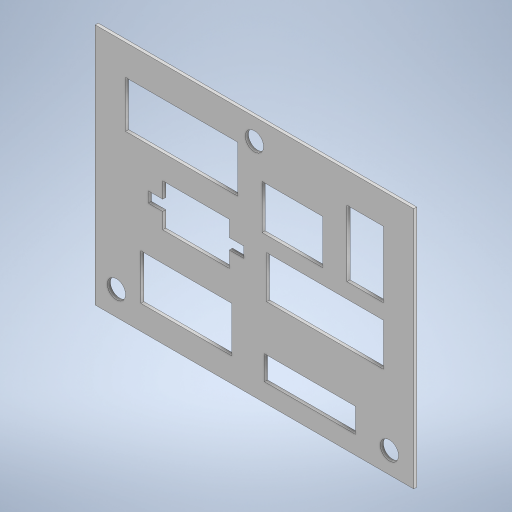
# Autodesk Inventor part: cap
Saved by Autodesk Inventor 2023 (Build 270158000, 158)
## iProperties
Created: 2023-04-07
Part Number: cap
Material: Generic
Document SubType Name: Sheet Metal
Designer: 310611102
Density: 1 g/cm^3
Sheet Metal Rule: Default_mm
Appearance: Default
Author: 310611102
Autodesk Inventor part; units mm, degrees
ref_plane "YZ Plane" through (0, 0, 0) normal (1, 0, 0) x (0, 1, 0)
ref_plane "XZ Plane" through (0, 0, 0) normal (0, 1, 0) x (-1, 0, 0)
ref_plane "XY Plane" through (0, 0, 0) normal (0, 0, 1) x (1, 0, 0)
sketch "Sketch1" plane through (0, 0, 0) normal (0, 0, 1) x (1, 0, 0)
  line L0 (-52.5, 40) -> (52.5, 40)
  line L1 (52.5, 40) -> (52.5, -40)
  line L2 (52.5, -40) -> (-52.5, -40)
  line L3 (-52.5, -40) -> (-52.5, 40)
  line L4 (-52.5, 40) -> (52.5, -40) construction
  line L5 (52.5, 40) -> (-52.5, -40) construction
  point P0 (0, 0)
  dimension "d0" = 80
  dimension "d1" = 105
  measures "d0" distance of L0.end L1.end
  measures "d1" distance of L0.start L0.end
extrude "Plate1" add sketch "Sketch1" along normal blind 1
sketch "Sketch3" plane through (0, 0, 0) normal (0, 0, -1) x (-1, 0, 0)
  line L0 (-42.5, 3.2) -> (-4, 3.2)
  line L1 (-4, 3.2) -> (-4, -10.8)
  line L2 (-4, -10.8) -> (-42.5, -10.8)
  line L3 (-42.5, -10.8) -> (-42.5, 3.2)
  line L4 (-42.5, 3.2) -> (-4, -10.8) construction
  line L5 (-4, 3.2) -> (-42.5, -10.8) construction
  line L6 (8.25, 6.6) -> (30.25, 6.6)
  line L7 (35, 1.35) -> (35, -2.15)
  line L8 (30.25, -7.4) -> (8.25, -7.4)
  line L9 (3.5, -2.15) -> (3.5, 1.35)
  line L10 (0.2073, 10) -> (38.2927, -10.8) construction
  line L11 (35, 6.6) -> (3.5, -7.4) construction
  line L12 (-2.5, 8.2) -> (-22.5, 8.2)
  line L13 (-22.5, 8.2) -> (-22.5, 22.8)
  line L14 (-22.5, 22.8) -> (-2.5, 22.8)
  line L15 (-2.5, 22.8) -> (-2.5, 8.2)
  line L16 (-2.5, 8.2) -> (-22.5, 22.8) construction
  line L17 (-22.5, 8.2) -> (-2.5, 22.8) construction
  line L18 (-3.29, -34) -> (-33.29, -34)
  line L19 (-33.29, -34) -> (-33.29, -26)
  line L20 (-33.29, -26) -> (-3.29, -26)
  line L21 (-3.29, -26) -> (-3.29, -34)
  line L22 (-3.29, -34) -> (-33.29, -26) construction
  line L23 (-33.29, -34) -> (-3.29, -26) construction
  line L24 (52.5, 40) -> (-52.5, 40) projected
  line L25 (52.5, -40) -> (52.5, 40) projected
  line L26 (30.25, -7.4) -> (30.25, -2.15)
  line L27 (30.25, -2.15) -> (35, -2.15)
  line L28 (30.25, 6.6) -> (30.25, 1.35)
  line L29 (30.25, 1.35) -> (35, 1.35)
  line L30 (8.25, -7.4) -> (8.25, -2.15)
  line L31 (8.25, -2.15) -> (3.5, -2.15)
  line L32 (8.25, 6.6) -> (8.25, 1.35)
  line L33 (8.25, 1.35) -> (3.5, 1.35)
  line L34 (-52.5, 40) -> (-52.5, -40) projected
  line L35 (-42.5, 30) -> (-30.5, 30)
  line L36 (-30.5, 30) -> (-30.5, 8.2)
  line L37 (-30.5, 8.2) -> (-42.5, 8.2)
  line L38 (-42.5, 8.2) -> (-42.5, 30)
  line L39 (7.5, -32) -> (37.5, -32)
  line L40 (37.5, -32) -> (37.5, -17)
  line L41 (37.5, -17) -> (7.5, -17)
  line L42 (7.5, -17) -> (7.5, -32)
  line L43 (-52.5, -40) -> (52.5, -40) projected
  point P0 (0, 0)
  point P1 (-23.25, -3.8)
  point P2 (19.25, -0.4)
  point P3 (-12.5, 15.5)
  point P4 (-18.29, -30)
  dimension "d14" = 14
  dimension "d17" = 7.5
  dimension "d22" = 20
  dimension "d24" = 14.6
  dimension "d37" = 8
  dimension "d40" = 30
  dimension "d46" = 17.2
  dimension "d47" = 55
  dimension "d48" = 17.5
  dimension "d49" = 33.4
  dimension "d50" = 66
  dimension "d65" = 14
  dimension "d66" = 31.5
  dimension "d67" = 3.5
  dimension "d68" = 22
  dimension "d69" = 5
  dimension "d70" = 10
  dimension "d71" = 10
  dimension "d72" = 10
  dimension "d73" = 8
  dimension "d74" = 5
  dimension "d75" = 19.21
  dimension "d76" = 15
  dimension "d77" = 8
  dimension "d78" = 15
  dimension "d79" = 30
  constraints: 80 end point, 12 parallel, 8 horizontal, 8 midpoint, 6 collinear, 6 perpendicular, 5 point on line, 2 vertical
  measures "d14" distance of L2.end L0.start
  measures "d17" distance between parallel lines of L1 L9
  measures "d22" distance of L12.start L12.end
  measures "d24" distance of L12.end L13.end
  measures "d37" distance of L20.end L18.start
  measures "d40" distance of L18.start L18.end
  measures "d46" distance between parallel lines of L24 L14
  measures "d47" distance between parallel lines of L25 L15
  measures "d48" distance between parallel lines of L25 L7
  measures "d49" distance between parallel lines of L24 L6
  measures "d50" distance between parallel lines of L24 L20
  measures "d65" distance between parallel lines of L6 L8
  measures "d66" distance between parallel lines of L9 L7
  measures "d67" distance of L9.start L9.end
  measures "d68" distance of L8.start L8.end
  measures "d69" distance between parallel lines of L12 L0
  measures "d70" distance between parallel lines of L34 L3
  measures "d71" distance between parallel lines of L34 L38
  measures "d72" distance between parallel lines of L24 L35
  measures "d73" distance between parallel lines of L13 L36
  measures "d74" distance between parallel lines of L0 L37
  measures "d75" distance between parallel lines of L19 L34
  measures "d76" distance between parallel lines of L25 L40
  measures "d77" distance between parallel lines of L43 L39
  measures "d78" distance of L41.end L39.start
  measures "d79" distance of L39.start L39.end
extrude "Extrusion1" cut sketch "Sketch3" against normal blind 10 contours L0 L1 L2 L3 | L6 L28 L29 L7 L27 L26 L8 L30 L31 L9 L33 L32 | L12 L13 L14 L15 | L18 L19 L20 L21 | L35 L36 L37 L38 | L42 L41 L40 L39
sketch "Sketch5" plane through (0, 0, 0) normal (0, 0, -1) x (-1, 0, 0)
  line L0 (42.5, 14.6) -> (5.5, 14.6)
  line L1 (5.5, 14.6) -> (5.5, 30)
  line L2 (5.5, 30) -> (42.5, 30)
  line L3 (42.5, 30) -> (42.5, 14.6)
  line L4 (42.5, 14.6) -> (5.5, 30) construction
  line L5 (5.5, 14.6) -> (42.5, 30) construction
  line L6 (8.25, 6.6) -> (30.25, 6.6) projected
  line L7 (-2.5, 22.8) -> (-2.5, 8.2) projected
  line L8 (-4, -10.8) -> (-42.5, -10.8) projected
  line L9 (52.5, 40) -> (-52.5, 40) projected
  line L10 (52.5, -40) -> (52.5, 40) projected
  point P0 (0, 0)
  point P1 (24, 22.3)
  point P2 (3.5, 1.6)
  point P3 (35, 1.6)
  point P4 (24, 14.6)
  dimension "d27" = 8
  dimension "d28" = 8
  dimension "d52" = 10
  dimension "d53" = 10
  constraints: 12 end point, 3 midpoint, 2 parallel, 1 horizontal, 1 perpendicular, 1 other
  measures "d28" distance between parallel lines of L7 L1
  measures "d52" distance between parallel lines of L9 L2
  measures "d53" distance between parallel lines of L10 L3
extrude "Extrusion2" cut sketch "Sketch5" against normal blind 10
sketch "Sketch7" plane through (0, 0, 0) normal (0, 0, -1) x (-1, 0, 0)
  point P0 (0, 0)
sketch "Sketch8" plane through (0, 0, 0) normal (0, 0, -1) x (-1, 0, 0)
  circle A0 centre (45.5, -32) radius 3
  circle A1 centre (-44.5, -33) radius 3
  circle A2 centre (0, 33) radius 3
  line L0 (52.5, -40) -> (52.5, 40) projected
  line L1 (-52.5, -40) -> (52.5, -40) projected
  line L2 (-52.5, 40) -> (-52.5, -40) projected
  line L3 (52.5, 40) -> (-52.5, 40) projected
  point P0 (0, 0)
  dimension "d54" = 6
  dimension "d55" = 6
  dimension "d56" = 6
  dimension "d57" = 7
  dimension "d58" = 8
  dimension "d60" = 8
  dimension "d61" = 7
  dimension "d62" = 7
  constraints: 3 centre point, 1 vertical alignment
  measures "d54" diameter of A0
  measures "d55" diameter of A1
  measures "d56" diameter of A2
  measures "d57" distance from line of L0 A0.centre
  measures "d58" distance from line of L1 A0.centre
  measures "d60" distance from line of L2 A1.centre
  measures "d61" distance from line of L1 A1.centre
  measures "d62" distance from line of L3 A2.centre
extrude "Extrusion3" cut sketch "Sketch8" against normal blind 10 contours A0 | A1 | A2
equation "\"d2\" = 厚度"
equation "\"折彎半徑\" = 厚度"
equation "\"最小剩餘\" = 2 * 厚度"
equation "\"轉移半徑\" = 折彎半徑"
equation "\"間隙大小\" = 厚度"
equation "\"折彎離隙寬度\" = 厚度"
equation "\"折彎離隙深度\" = 0.5 * 厚度"
equation "\"轉角離隙大小\" = 4 * 厚度"
equation "\"Jacobi半徑大小\" = 折彎半徑"
equation "\"厚度\" = 1"
body "Solid1"
